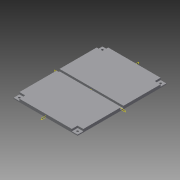
# Autodesk Inventor part: transillum_diffusor_partC_v1
Saved by Autodesk Inventor 2015 (Build 190159000, 159)
## iProperties
Created: 2022-05-26
Part Number: transillum_diffusor_partC_v1
Material: Genérico
Document SubType Name: Modeling
Designer: Zuloaga
Density: 1 g/cm^3
Appearance: Valor por defecto
Author: Zuloaga
Autodesk Inventor part; units mm, degrees
ref_plane "YZ Plane" through (0, 0, 0) normal (1, 0, 0) x (0, 1, 0)
ref_plane "XZ Plane" through (0, 0, 0) normal (0, 1, 0) x (-1, 0, 0)
ref_plane "XY Plane" through (0, 0, 0) normal (0, 0, 1) x (1, 0, 0)
sketch "Boceto1" plane through (0, 0, 0) normal (0, 0, 1) x (1, 0, 0)
  line L0 (0, 0) -> (127.5, 0)
  line L1 (127.5, 0) -> (127.5, 177)
  line L2 (127.5, 177) -> (0, 177)
  line L3 (0, 177) -> (0, 0)
  dimension "d32" = 127.5
  dimension "d33" = 177
  constraints: 8 end point, 2 parallel, 1 horizontal, 1 perpendicular
  measures "d32" distance of L2.end L1.end
  measures "d33" distance of L1.end L0.end
extrude "Extrusión1" add sketch "Boceto1" along normal blind 6
ref_plane "Plano de trabajo6" through (0, 88.5, 0) normal (0, -1, 0) x (1, 0, 0)
ref_plane "Plano de trabajo7" through (63.75, 0, 0) normal (-1, 0, 0) x (0, 0, 1)
sketch "Boceto17" plane through (0, 0, 6) normal (0, 0, 1) x (1, 0, 0)
  line L0 (127.5, 0) -> (116, 0)
  line L1 (116, 0) -> (116, 11.5)
  line L2 (116, 11.5) -> (127.5, 11.5)
  line L3 (127.5, 11.5) -> (127.5, 0)
  line L4 (0, 0) -> (11.5, 0)
  line L5 (11.5, 0) -> (11.5, 11.5)
  line L6 (11.5, 11.5) -> (0, 11.5)
  line L7 (0, 11.5) -> (0, 0)
  line L8 (127.5, 177) -> (116, 177)
  line L9 (116, 177) -> (116, 165.5)
  line L10 (116, 165.5) -> (127.5, 165.5)
  line L11 (127.5, 165.5) -> (127.5, 177)
  line L12 (0, 177) -> (11.5, 177)
  line L13 (11.5, 177) -> (11.5, 165.5)
  line L14 (11.5, 165.5) -> (0, 165.5)
  line L15 (0, 165.5) -> (0, 177)
  dimension "d124" = 11.5
  dimension "d125" = 11.5
  dimension "d129" = 11.5
  dimension "d130" = 11.5
  dimension "d131" = 11.5
  dimension "d132" = 11.5
  dimension "d133" = 11.5
  dimension "d134" = 11.5
  constraints: 32 end point, 8 parallel, 4 horizontal, 4 perpendicular
  measures "d124" distance of L1.end L2.end
  measures "d125" distance of L0.end L1.end
  measures "d129" distance of L6.end L5.end
  measures "d130" distance of L5.end L4.end
  measures "d131" distance of L10.end L9.end
  measures "d132" distance of L9.end L8.end
  measures "d133" distance of L13.end L14.end
  measures "d134" distance of L12.end L13.end
extrude "Extrusión12" cut sketch "Boceto17" against normal blind 4
sketch "Boceto18" plane through (0, 0, 2) normal (0, 0, 1) x (1, 0, 0)
  line L0 (0, 0) -> (11.5, 0)
  line L1 (11.5, 0) -> (11.5, 11.5)
  line L2 (11.5, 11.5) -> (0, 11.5)
  line L3 (0, 11.5) -> (0, 0)
  line L4 (127.5, 0) -> (116, 0)
  line L5 (116, 0) -> (116, 11.5)
  line L6 (116, 11.5) -> (127.5, 11.5)
  line L7 (127.5, 11.5) -> (127.5, 0)
  line L8 (127.5, 177) -> (116, 177)
  line L9 (116, 177) -> (116, 165.5)
  line L10 (116, 165.5) -> (127.5, 165.5)
  line L11 (127.5, 165.5) -> (127.5, 177)
  line L12 (0, 177) -> (11.5, 177)
  line L13 (11.5, 177) -> (11.5, 165.5)
  line L14 (11.5, 165.5) -> (0, 165.5)
  line L15 (0, 165.5) -> (0, 177)
  line L16 (116, 11.5) -> (127.5, 0)
  line L17 (127.5, 11.5) -> (116, 0)
  circle A0 centre (121.75, 5.75) radius 2
  dimension "d137" = 4
  constraints: 36 end point, 8 parallel, 5 perpendicular, 4 horizontal, 2 point on line, 1 centre point, 1 midpoint
  measures "d137" diameter of A0
extrude "Extrusión13" cut sketch "Boceto18" against normal blind 3.2 contours A0 L17 L16 | L16 L17 A0 | A0 L16 L17 | L17 L16 A0
mirror "Simetría7" about plane through (63.75, 0, 0) normal (-1, 0, 0) of "Extrusión13"
mirror "Simetría8" about plane through (0, 88.5, 0) normal (0, -1, 0) of "Extrusión13", "Simetría7"
sketch "Boceto19" plane through (0, 0, 6) normal (0, 0, 1) x (1, 0, 0)
  line L0 (0, 0) -> (127.5, 0)
  line L1 (127.5, 0) -> (127.5, 85.5)
  line L2 (127.5, 85.5) -> (0, 85.5)
  line L3 (0, 85.5) -> (0, 0)
  line L4 (127.5, 0) -> (127.5, 177) projected
  line L5 (0, 85.5) -> (127.5, 85.5)
  line L6 (127.5, 85.5) -> (127.5, 91.5)
  line L7 (127.5, 91.5) -> (0, 91.5)
  line L8 (0, 91.5) -> (0, 85.5)
  line L9 (0, 91.5) -> (127.5, 91.5)
  line L10 (127.5, 91.5) -> (127.5, 177)
  line L11 (127.5, 177) -> (0, 177)
  line L12 (0, 177) -> (0, 91.5)
  dimension "d140" = 127.5
  dimension "d141" = 85.5
  dimension "d142" = 6
  constraints: 24 end point, 6 parallel, 3 horizontal, 3 perpendicular, 1 point on line
  measures "d140" distance of L2.end L1.end
  measures "d141" distance of L1.end L0.end
  measures "d142" distance of L6.end L5.end
extrude "Extrusión14" cut sketch "Boceto19" against normal blind 4.2 contours L8 L7 L4 L2
